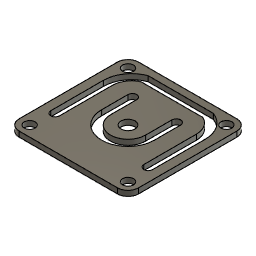
T-Puck_V3 (Autodesk Fusion 360 archive; units mm, degrees)
design "Wägezelle"
Autodesk Fusion 360 part; units mm, degrees
sketch "Skizze1" plane through (0, 0, 0) normal (0, 1, 0) x (1, 0, 0)
  line L0 (-17, 17) -> (17, 17)
  line L1 (17, 17) -> (17, -17)
  line L2 (17, -17) -> (-17, -17)
  line L3 (-17, -17) -> (-17, 17)
  line L4 (0, 0) -> (0, 17) construction
  line L5 (0, 0) -> (17, 0) construction
  circle A0 centre (0, 0) radius 2
  circle A1 centre (-14, 14) radius 1.55
  circle A2 centre (14, 14) radius 1.55
  circle A3 centre (-14, -14) radius 1.55
  circle A4 centre (14, -14) radius 1.55
  circle A5 centre (0, 0) radius 5
  circle A6 centre (-13.25, -7.5) radius 1.25
  line L6 (-12, -7.5) -> (-12, 7.5)
  line L7 (-14.5, -7.5) -> (-14.5, 7.5)
  circle A7 centre (-6.5, 7.5) radius 5.5
  circle A8 centre (-6.5, 7.5) radius 8
  line L8 (-9.2839, 15) -> (0, 15)
  line L9 (-8.7913, 12.5) -> (0, 12.5)
  circle A9 centre (6.5, 7.5) radius 8
  circle A10 centre (6.5, 7.5) radius 5.5
  line L10 (8.7913, 12.5) -> (0, 12.5)
  line L11 (9.2839, 15) -> (0, 15)
  line L12 (12, -7.5) -> (12, 7.5)
  line L13 (14.5, -7.5) -> (14.5, 7.5)
  circle A11 centre (13.25, -7.5) radius 1.25
  dimension "d1" = 34
  dimension "d7" = 4
  dimension "d11" = 3.1
  dimension "d12" = 28
  dimension "d13" = 28
  dimension "d14" = 10
  dimension "d17" = 2.5
  dimension "d18" = 2.5
  dimension "d20" = 16
  dimension "d21" = 11
  dimension "d22" = 9.5
  dimension "d23" = 2
  dimension "d24" = 2.5
  dimension "d28" = 9.5
  constraint horizontal L0
  constraint vertical L1
  constraint horizontal L2
  constraint vertical L3
  constraint coincident L4.start L5.start
  constraint midpoint L0 L4.end
  constraint midpoint L1 L5.end
  constraint horizontal L5
  constraint vertical L4
  constraint equal L0 L1
  constraint symmetric L4 A1 A2
  constraint symmetric L5 A1 A3
  constraint symmetric L5 A2 A4
  constraint coincident A6 L6.start
  constraint tangent A6 L6
  constraint vertical L6
  constraint coincident A6 L7.start
  constraint tangent A6 L7
  constraint parallel L6 L7
  constraint concentric A7 A8
  constraint tangent L7 A8
  constraint coincident L7.end A8
  constraint coincident L6.end A7
  constraint coincident A8 L8.start
  constraint coincident L4 L8.end
  constraint perpendicular L4 L8
  constraint coincident A7 L9.start
  constraint coincident L4 L9.end
  constraint perpendicular L4 L9
  constraint symmetric L4 A6 A11
  constraint symmetric L4 L6.start L12.start
  constraint symmetric L4 L6.end L12.end
  constraint symmetric L4 L7.start L13.start
  constraint symmetric L4 L7.end L13.end
  constraint symmetric L4 A7 A10
  constraint symmetric L4 A8 A9
  constraint symmetric L4 L8.start L11.start
  constraint symmetric L4 L8.end L11.end
  constraint symmetric L4 L9.start L10.start
  constraint symmetric L4 L9.end L10.end
  measures "d1" distance of L0.start L0.end
  measures "d7" diameter of A0
  measures "d11" diameter of A1
  measures "d12" distance of A1.centre A2.centre
  measures "d13" distance of A2.centre A4.centre
  measures "d14" diameter of A5
  measures "d17" distance of L3 L7
  measures "d18" distance of L6 L7
  measures "d20" diameter of A8
  measures "d21" diameter of A7
  measures "d22" distance of L2 A6.centre
  measures "d23" distance of L0 L8
  measures "d24" distance of L8 L9
  measures "d28" distance of L0 A7.centre
extrude "Extrusion1" add sketch "Skizze1" along normal blind 1.5 contours L0 L1 L2 L3 | A0 A5 A8 A9 | A0 A5 A8 A9 A10 | A0 A5 A7 A8 A9 | A0 A8 A9 | A5 A9 A10 L12 | A5 L6 A7 A8 | A5 A8 A9 | A9 A10 L10 L11 L12 | A9 L12 L13 A11 | A5 A7 L9 A9 | A5 A7 | L6 A7 A8 L8 L9 | A6 L6 L7 A8 | A5 A8 A10 | A5 A7 A8 A9 A10 | A5 A7 A9 | A5 A10 | A5 A8 A10 L10 | A11 | A6 | A8 A10 | A7 A9 | A9 L11 | A10 L10 | A7 L9 | A8 L8 | A8 A9 A10 L10 | A7 A8 L9 A9 | A8 L8 L9 A9 L10 L11 | A8 L9 A9 L10 picked at (0.0445, 2.311)
fillet "Abrundung1" radius 3 4 edges at (-17, 0.75, -17) (-17, 0.75, 17) (17, 0.75, 17) (17, 0.75, -17)
extrude "Extrusion2" cut sketch "Skizze1" along normal up to surface (1.5 mm away) contours A9 A10 L10 L11 L12 | A9 L12 L13 A11 | L6 A7 A8 L8 L9 | A6 L6 L7 A8 | A11 | A6 | A10 L10 | A7 L9 | A8 L8 L9 A9 L10 L11
sketch "Skizze2" plane through (0, 0, 0) normal (0, -1, 0) x (1, 0, 0)
  arc A0 (-12, 7.5) -> (-14.5, 7.5) centre (-13.25, 7.5) ccw
  line L0 (-12, 7.5) -> (-12, -7.5)
  arc A1 (-12, -7.5) -> (-8.7913, -12.5) centre (-6.5, -7.5) ccw
  line L1 (-8.7913, -12.5) -> (8.7913, -12.5)
  arc A2 (8.7913, -12.5) -> (12, -7.5) centre (6.5, -7.5) ccw
  line L2 (12, -7.5) -> (12, 7.5)
  arc A3 (14.5, 7.5) -> (12, 7.5) centre (13.25, 7.5) ccw
  line L3 (14.5, 7.5) -> (14.5, -7.5)
  arc A4 (9.2839, -15) -> (14.5, -7.5) centre (6.5, -7.5) ccw
  line L4 (9.2839, -15) -> (-9.2839, -15)
  arc A5 (-14.5, -7.5) -> (-9.2839, -15) centre (-6.5, -7.5) ccw
  line L5 (-14.5, -7.5) -> (-14.5, 7.5)
  circle A6 centre (-14, 14) radius 1.55
  circle A7 centre (14, -14) radius 1.55
  circle A8 centre (14, 14) radius 1.55
  circle A9 centre (-14, -14) radius 1.55
  circle A10 centre (0, 0) radius 2
  arc A11 (14, -17) -> (17, -14) centre (14, -14) ccw
  line L6 (17, -14) -> (17, 14)
  arc A12 (17, 14) -> (14, 17) centre (14, 14) ccw
  line L7 (14, 17) -> (-14, 17)
  arc A13 (-14, 17) -> (-17, 14) centre (-14, 14) ccw
  line L8 (-17, 14) -> (-17, -14)
  arc A14 (-17, -14) -> (-14, -17) centre (-14, -14) ccw
  line L9 (-14, -17) -> (14, -17)
  circle A15 centre (0, 0) radius 5
  line L10 (0, 0) -> (0, -17) construction
  circle A16 centre (6.25, -7.5) radius 1.25
  line L11 (5, 0) -> (5, -7.5)
  line L12 (7.5, -7.5) -> (7.5, 0)
  circle A17 centre (0, 0) radius 7.5
  line L13 (0, 0) -> (7.5, 0) construction
  circle A18 centre (-6.25, -7.5) radius 1.25
  line L14 (-5, 0) -> (-5, -7.5)
  line L15 (-7.5, -7.5) -> (-7.5, 0)
  dimension "d31" = 2.5
  dimension "d32" = 10
  dimension "d33" = 7.5
  constraint concentric A10 A15
  constraint coincident A10.centre A15.centre
  constraint midpoint L9 L10.end
  constraint coincident A15 L11.start
  constraint coincident A16 L11.end
  constraint tangent A16 L11
  constraint vertical L11
  constraint coincident A16 L12.start
  constraint tangent A16 L12
  constraint parallel L11 L12
  constraint concentric A15 A17
  constraint coincident L12.end A17
  constraint tangent L12 A17
  constraint tangent A15 L11
  constraint symmetric L10 A16 A18
  constraint symmetric L10 L11.start L14.start
  constraint symmetric L10 L11.end L14.end
  constraint symmetric L10 L12.start L15.start
  constraint symmetric L10 L12.end L15.end
  measures "d31" distance of L11 L12
  measures "d32" diameter of A15
  measures "d33" distance of A16.centre L13
extrude "Extrusion3" cut sketch "Skizze2" against normal up to surface (1.5 mm away) contours A15 L11 A17 L14 | A16 L11 L12 A17 | A17 A18 L14 L15 | A16 | A18 picked at (-4.6131, 4.7886)
equation "d13 = d12"
equation "d21 = d20 - 5 mm"

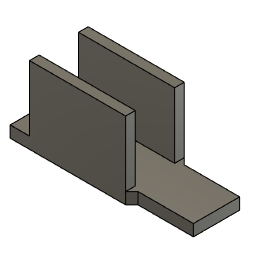
design "nRF52840-Dongle"
Autodesk Fusion 360 part; units mm, degrees
sketch "Skizze1" plane through (0, 0, 0) normal (0, 1, 0) x (1, 0, 0)
  line L0 (-15.015, 0) -> (31.025, 0) construction
  line L1 (-15.015, 0) -> (-15.015, -7.62)
  line L2 (-15.015, -7.62) -> (15.015, -7.62)
  line L3 (15.015, -7.62) -> (16.625, -6.01)
  line L4 (16.625, -6.01) -> (31.025, -6.01)
  line L5 (31.025, -6.01) -> (31.025, 0)
  line L6 (-15.015, 0) -> (-15.015, 7.62)
  line L7 (-15.015, 7.62) -> (15.015, 7.62)
  line L8 (15.015, 7.62) -> (16.625, 6.01)
  line L9 (16.625, 6.01) -> (31.025, 6.01)
  line L10 (31.025, 6.01) -> (31.025, 0)
  line L11 (0, 0) -> (0, 7.62) construction
  dimension "d1" = 12.02
  dimension "d2" = 15.24
  dimension "d3" = 30.03
  dimension "d4" = 14.4
  dimension "d5" = 46.04
  constraint horizontal L0
  constraint perpendicular L0 L1
  constraint perpendicular L1 L2
  constraint parallel L0 L4
  constraint perpendicular L0 L5
  constraint symmetric L1.start L0 L6.start
  constraint symmetric L5.end L0 L10.end
  constraint symmetric L0 L1.end L6.end
  constraint symmetric L0 L2.end L7.end
  constraint symmetric L0 L3.end L8.end
  constraint symmetric L0 L4.end L9.end
  constraint coincident L11.start origin
  constraint midpoint L7 L11.end
  constraint vertical L11
  constraint coincident L11.start L0
  measures "d1" distance of L4 L9
  measures "d2" distance of L2 L7
  measures "d3" distance of L1.end L2.end
  measures "d4" distance of L3.end L4.end
  measures "d5" distance of L1 L5
extrude "Extrusion1" add sketch "Skizze1" along normal blind 3
sketch "Skizze2" plane through (0, 3, 0) normal (0, 1, 0) x (-1, 0, 0)
  line L0 (15.015, -7.62) -> (15.015, 7.62)
  line L1 (15.015, 7.62) -> (-15.015, 7.62)
  line L2 (-15.015, 7.62) -> (-16.625, 6.01)
  line L3 (-16.625, 6.01) -> (-31.025, 6.01)
  line L4 (-31.025, 6.01) -> (-31.025, -6.01)
  line L5 (-31.025, -6.01) -> (-16.625, -6.01)
  line L6 (-16.625, -6.01) -> (-15.015, -7.62)
  line L7 (-15.015, -7.62) -> (15.015, -7.62)
  line L8 (9.985, 5.12) -> (-15.015, 5.12)
  line L9 (-15.015, 5.12) -> (-15.015, 7.62)
  line L10 (-15.015, 7.62) -> (9.985, 7.62)
  line L11 (9.985, 7.62) -> (9.985, 5.12)
  line L12 (0, 0) -> (-10, 0) construction
  line L13 (-15.015, -7.62) -> (9.985, -7.62)
  line L14 (9.985, -7.62) -> (9.985, -5.12)
  line L15 (-15.015, -5.12) -> (-15.015, -7.62)
  line L16 (9.985, -5.12) -> (-15.015, -5.12)
  dimension "d8" = 25
  dimension "d9" = 2.5
  constraint horizontal L8
  constraint vertical L9
  constraint horizontal L10
  constraint vertical L11
  constraint coincident L1 L2.start
  constraint coincident L1.end L2.start
  constraint coincident L12.start origin
  constraint horizontal L12
  constraint symmetric L8.start L12 L14.end
  constraint symmetric L8.end L12 L15.start
  constraint symmetric L1.end L12 L6.end
  constraint symmetric L10.end L12 L13.end
  measures "d8" distance of L1.end L10.end
  measures "d9" distance of L8.start L10.end
extrude "Extrusion2" add sketch "Skizze2" along normal blind 17 contours L7 L13 L14 L15 L16 | L1 L8 L9 L10 L11

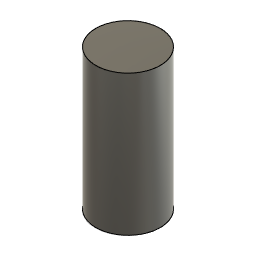
design "Battery"
Autodesk Fusion 360 part; units mm, degrees
sketch "Skizze1" plane through (0, 0, 0) normal (0, 1, 0) x (1, 0, 0)
  circle A0 centre (0, 0) radius 8.25
  dimension "d1" = 16.5
  constraint coincident A0.centre origin
  measures "d1" diameter of A0
extrude "Extrusion1" add sketch "Skizze1" along normal blind 36

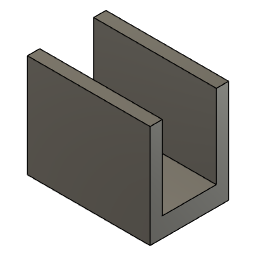
design "ADC_Wägezelle"
Autodesk Fusion 360 part; units mm, degrees
sketch "Skizze1" plane through (0, 0, 0) normal (0, 1, 0) x (1, 0, 0)
  line L0 (-12.5, 8) -> (12.5, 8)
  line L1 (12.5, 8) -> (12.5, -8)
  line L2 (12.5, -8) -> (-12.5, -8)
  line L3 (-12.5, -8) -> (-12.5, 8)
  line L4 (0, 0) -> (0, 8) construction
  line L5 (0, 0) -> (12.5, 0) construction
  dimension "d1" = 25
  dimension "d2" = 16
  constraint horizontal L0
  constraint vertical L1
  constraint horizontal L2
  constraint vertical L3
  constraint coincident L4.start L5.start
  constraint midpoint L0 L4.end
  constraint midpoint L1 L5.end
  constraint vertical L4
  constraint horizontal L5
  measures "d1" distance of L0.start L0.end
  measures "d2" distance of L0.start L2.end
extrude "Extrusion1" add sketch "Skizze1" along normal blind 4
sketch "Skizze2" plane through (0, 4, 0) normal (0, 1, 0) x (-1, 0, 0)
  line L0 (12.5, 8) -> (-12.5, 8)
  line L1 (-12.5, 8) -> (-12.5, -8)
  line L2 (-12.5, -8) -> (12.5, -8)
  line L3 (12.5, -8) -> (12.5, 8)
  line L4 (12.5, 8) -> (-12.5, 8)
  line L5 (-12.5, 8) -> (-12.5, 5.5)
  line L6 (-12.5, 5.5) -> (12.5, 5.5)
  line L7 (12.5, 5.5) -> (12.5, 8)
  line L8 (0, 0) -> (-10, 0) construction
  line L9 (12.5, -8) -> (-12.5, -8)
  line L10 (-12.5, -8) -> (-12.5, -5.5)
  line L11 (-12.5, -5.5) -> (12.5, -5.5)
  line L12 (12.5, -5.5) -> (12.5, -8)
  dimension "d5" = 2.5
  constraint horizontal L4
  constraint vertical L5
  constraint horizontal L6
  constraint vertical L7
  constraint coincident L0 L3.end
  constraint coincident L0.start L3.end
  constraint coincident L0.end L1.start
  constraint coincident L8.start origin
  constraint horizontal L8
  constraint symmetric L0.start L8 L2.end
  constraint symmetric L0.end L8 L1.end
  constraint symmetric L5.end L8 L10.end
  constraint symmetric L6.end L8 L11.end
  measures "d5" distance of L0.end L5.end
extrude "Extrusion2" add sketch "Skizze2" along normal blind 17 contours L0 L1 L3 L4 L5 L6 L7 | L1 L2 L3 L9 L10 L11 L12
